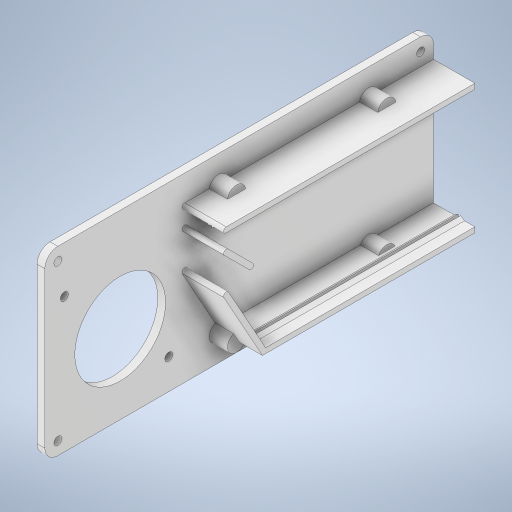
# Autodesk Inventor part: ChargingCircuit - ShroudPlate - Version2
Saved by Autodesk Inventor 2023 (Build 270158000, 158)
## iProperties
Created: 2023-01-17
Part Number: ChargingCircuit - ShroudPlate - Version2
Material: ABS Plastic
Document SubType Name: Modeling
Designer: ethan
Density: 1.06 g/cm^3
Appearance: Smooth - White
Author: ethan
Autodesk Inventor part; units mm, degrees
ref_plane "YZ Plane" through (0, 0, 0) normal (1, 0, 0) x (0, 1, 0)
ref_plane "XZ Plane" through (0, 0, 0) normal (0, 1, 0) x (-1, 0, 0)
ref_plane "XY Plane" through (0, 0, 0) normal (0, 0, 1) x (1, 0, 0)
sketch "Sketch1" plane through (0, 0, 0) normal (0, 0, 1) x (1, 0, 0)
  line L0 (0, 0) -> (150, 0)
  line L1 (150, 0) -> (150, 70)
  line L2 (150, 70) -> (0, 70)
  line L3 (0, 70) -> (0, 0)
  line L4 (5, 65) -> (145, 65) construction
  line L5 (145, 5) -> (5, 5) construction
  line L6 (5, 5) -> (5, 65) construction
  circle A0 centre (5, 65) radius 1.5
  circle A1 centre (5, 5) radius 1.5
  circle A2 centre (145, 5) radius 1.5
  circle A3 centre (145, 65) radius 1.5
  line L7 (102.1949, 52) -> (142.5, 52) construction
  line L8 (142.5, 52) -> (142.5, 11.6949) construction
  line L9 (142.5, 11.6949) -> (102.1949, 11.6949) construction
  line L10 (102.1949, 11.6949) -> (102.1949, 52) construction
  circle A4 centre (102.1949, 11.6949) radius 1.5
  circle A5 centre (142.5, 52) radius 1.5
  line L11 (102.1949, 11.6949) -> (142.5, 52) construction
  circle A6 centre (120.9332, 30.4332) radius 17.5
  line L12 (144, 53.5) -> (100.6949, 53.5) construction
  line L13 (100.6949, 53.5) -> (100.6949, 10.1949) construction
  line L14 (100.6949, 10.1949) -> (144, 10.1949) construction
  line L15 (144, 10.1949) -> (144, 53.5) construction
  line L16 (0, 56.6525) -> (0, 58.6525)
  line L17 (100.6949, 53.5) -> (100.6949, 35.6525) construction
  dimension "d0" = 150
  dimension "d1" = 70
  dimension "d2" = 5
  dimension "d3" = 5
  dimension "d4" = 60
  dimension "d5" = 140
  dimension "d6" = 3
  dimension "d7" = 3
  dimension "d8" = 3
  dimension "d9" = 3
  dimension "d13" = 40.3051
  dimension "d14" = 40.3051
  dimension "d15" = 3
  dimension "d16" = 3
  dimension "d18" = 35
  dimension "d48" = 18
  dimension "d49" = 7.5
  dimension "d50" = 18.7383
  constraints: 36 end point, 7 centre point, 7 parallel, 6 coincident, 4 horizontal, 4 tangent, 3 perpendicular, 3 point on line
  measures "d0" distance of L2.end L1.end
  measures "d1" distance of L1.end L0.end
  measures "d2" distance between parallel lines of L2 L4
  measures "d3" distance between parallel lines of L3 L6
  measures "d4" distance of L4.end L5.start
  measures "d5" distance of L4.start L4.end
  measures "d6" diameter of A0
  measures "d7" diameter of A1
  measures "d8" diameter of A2
  measures "d9" diameter of A3
  measures "d13" distance of L9.end L7.start
  measures "d14" distance of L7.start L7.end
  measures "d15" diameter of A4
  measures "d16" diameter of A5
  measures "d18" diameter of A6
  measures "d48" distance from line of L11.end L2
  measures "d49" distance from line of L1 L7.end
  measures "d50" horizontal distance of A6.centre L9.end
extrude "Extrusion1" add sketch "Sketch1" along normal blind 3
fillet "Fillet1" radius 5 4 edges at (0, 70, 1.5) (0, 0, 1.5) (150, 0, 1.5) (150, 70, 1.5)
sketch "Sketch2" plane through (0, 0, 0) normal (0, 0, -1) x (-1, 0, 0)
  line L0 (-150, 60) -> (-97, 60)
  line L1 (-150, 5) -> (-150, 65) projected
  line L2 (0, 65) -> (0, 5) projected
  line L3 (-145, 70) -> (-5, 70) projected
  line L4 (-97, 60) -> (-97, 0)
  line L5 (-5, 0) -> (-145, 0) projected
  line L6 (-97, 37) -> (-82, 10)
  line L7 (-82, 10) -> (0, 10)
  line L8 (0, 65) -> (0, 5) projected
  line L9 (-97, 41.1183) -> (-80.8232, 12)
  line L10 (-80.8232, 12) -> (0, 12)
  line L11 (-97, 60) -> (0, 60)
  line L12 (-97, 58) -> (0, 58)
  line L13 (0, 60) -> (0, 58)
  line L14 (0, 12) -> (0, 10)
  line L15 (-97, 51.1183) -> (-86.3934, 40.5117)
  line L16 (-97, 53.9467) -> (-84.9792, 41.9259)
  line L17 (-86.3934, 40.5117) -> (-84.9792, 41.9259)
  point P0 (0, 0)
  point P1 (0, 12)
  point P2 (0, 10)
  point P3 (-98, 58)
  point P4 (0, 58)
  dimension "d31" = 10
  dimension "d32" = 53
  dimension "d33" = 23
  dimension "d35" = 15
  dimension "d36" = 10
  dimension "d37" = 2
  dimension "d38" = 2
  dimension "d41" = 2
  dimension "d44" = 10
  dimension "d51" = 15
  dimension "d52" = 45
  dimension "d72" = 2
  constraints: 26 end point, 9 point on line, 3 horizontal, 3 parallel, 2 perpendicular, 2 vertical
  measures "d31" distance between parallel lines of L0 L3
  measures "d32" distance between parallel lines of L4 L1
  measures "d33" distance from line of L0 L6.start
  measures "d35" distance from line of L4 L6.end
  measures "d36" distance between parallel lines of L5 L7
  measures "d37" distance between parallel lines of L6 L9
  measures "d38" distance between parallel lines of L11 L12
  measures "d41" distance between parallel lines of L7 L10
  measures "d44" distance of L9.start L15.start
  measures "d51" distance of L15.start L15.end
  measures "d52" angle of L15 L4
  measures "d72" distance between parallel lines of L16 L15
extrude "Extrusion3" add sketch "Sketch2" along normal blind 16 contours L2 L12 L4 L11 | L2 L7 L6 L4 L9 L10 | L16 L17 L15 L4
fillet "Fillet2" radius 1 8 edges at (97, 41.1183, -8) (97, 60, -8) (97, 58, -8) (97, 37, -8) (97, 51.1183, -8) (97, 53.9467, -8) (84.9792, 41.9259, -8) (86.3934, 40.5117, -8)
sketch "Sketch3" plane through (0, 0, 3) normal (0, 0, 1) x (1, 0, 0)
  line L0 (25, 59.5) -> (83, 59.5) construction
  line L1 (83, 59.5) -> (83, 10.5) construction
  line L2 (83, 10.5) -> (25, 10.5) construction
  line L3 (25, 10.5) -> (25, 59.5) construction
  line L4 (5, 0) -> (145, 0) construction
  line L5 (145, 70) -> (5, 70) construction
  line L6 (1.5, 63) -> (86.5, 63) construction
  line L7 (86.5, 63) -> (86.5, 7) construction
  line L8 (86.5, 7) -> (1.5, 7) construction
  line L9 (1.5, 7) -> (1.5, 63) construction
  circle A0 centre (25, 10.5) radius 1.25
  circle A1 centre (25, 59.5) radius 1.25
  circle A2 centre (83, 59.5) radius 1.25
  circle A3 centre (83, 10.5) radius 1.25
  line L10 (0, 65) -> (0, 5) projected
  circle A4 centre (25, 59.5) radius 3.5
  circle A5 centre (83, 59.5) radius 3.5
  circle A6 centre (83, 10.5) radius 3.5
  circle A7 centre (25, 10.5) radius 3.5
  point P0 (0, 0)
  dimension "d53" = 58
  dimension "d54" = 49
  dimension "d55" = 70
  dimension "d56" = 10.5
  dimension "d57" = 85
  dimension "d58" = 56
  dimension "d59" = 3.5
  dimension "d61" = 2.5
  dimension "d62" = 2.5
  dimension "d63" = 2.5
  dimension "d64" = 2.5
  dimension "d70" = 1.5
  dimension "d71" = 3.5
  constraints: 16 end point, 8 centre point, 8 coincident, 4 parallel, 4 tangent, 2 horizontal, 2 perpendicular
  measures "d53" distance of L1.end L2.end
  measures "d54" distance of L0.end L1.end
  measures "d55" distance between parallel lines of L4 L5
  measures "d56" distance between parallel lines of L5 L0
  measures "d57" distance of L7.end L8.end
  measures "d58" distance of L6.end L7.end
  measures "d59" distance between parallel lines of L0 L6
  measures "d61" diameter of A0
  measures "d62" diameter of A1
  measures "d63" diameter of A2
  measures "d64" diameter of A3
  measures "d70" distance between parallel lines of L10 L9
  measures "d71" distance from line of L7 A3.centre
extrude "Extrusion5" add sketch "Sketch3" against normal blind 10 contours A0 | A1 | A2 | A3 | A4 | A5 | A6 | A7
extrude "Extrusion4" cut sketch "Sketch3" against normal blind 7 contours A0 | A1 | A2 | A3
sketch "Sketch4" plane through (0, 5, 3) normal (-1, 0, 0) x (0, 0, 1)
  line L0 (-3, 53) -> (-19, 53) projected
  line L1 (-3, 7) -> (-19, 7) projected
  line L2 (-12.5, 7) -> (-12.5, 8)
  line L3 (-12.5, 8) -> (-11, 7)
  line L4 (-13.5, 7) -> (-13.5, 8)
  line L5 (-13.5, 8) -> (-15, 7)
  line L6 (-11, 53) -> (-12.5, 53)
  line L7 (-12.5, 52) -> (-11, 53)
  line L8 (-12.5, 53) -> (-12.5, 52)
  line L9 (-13.5, 53) -> (-13.5, 52)
  line L10 (-13.5, 52) -> (-15, 53)
  line L11 (-13.5, 53) -> (-15, 53)
  line L12 (-12.5, 53) -> (-11, 53)
  line L13 (-15, 7) -> (-13.5, 7)
  line L14 (-12.5, 7) -> (-11, 7)
  point P0 (-3, -5)
  dimension "d73" = 1
  dimension "d74" = 1.5
  dimension "d75" = 1.5
  dimension "d76" = 1
  dimension "d77" = 1
  dimension "d78" = 1
  dimension "d79" = 1
  dimension "d80" = 1.5
  dimension "d81" = 1.5
  dimension "d82" = 1
  constraints: 26 end point, 4 collinear, 4 midpoint, 4 point on line, 3 vertical, 1 perpendicular
  measures "d73" distance of L2.start L2.end
  measures "d74" distance of L14.end L2.start
  measures "d75" distance of L5.end L4.start
  measures "d76" distance of L4.start L2.start
  measures "d77" distance of L6.end L8.end
  measures "d78" distance of L9.start L9.end
  measures "d79" distance of L9.start L6.end
  measures "d80" distance of point (-11, 53) L6.end
  measures "d81" distance of L10.end L9.start
  measures "d82" distance of L4.start L4.end
extrude "Extrusion6" add sketch "Sketch4" against normal up to surface contours L1 L2 L3 | L1 L5 L4 surface through (80.8232, 12, 0) normal (-0.8741573, 0.4856429, 0)
sketch "Sketch5" plane through (0, 5, 3) normal (-1, 0, 0) x (0, 0, 1)
  line L0 (-11, 7) -> (-12.5, 8) projected
  line L1 (-11, 7) -> (-11, 53)
  line L2 (-3, 53) -> (-19, 53) projected
  line L3 (-11, 53) -> (-12.5, 53)
  line L4 (-12.5, 53) -> (-12.5, 52)
  line L5 (-12.5, 52) -> (-11, 53)
  line L6 (-12.5, 53) -> (-13.5, 53)
  line L7 (-13.5, 53) -> (-13.5, 52)
  line L8 (-13.5, 52) -> (-15, 53)
  line L9 (-15, 53) -> (-13.5, 53)
  point P0 (-3, -5)
  dimension "d85" = 1.5
  dimension "d86" = 1
  dimension "d87" = 1
  dimension "d88" = 1.5
  dimension "d89" = 1
  constraints: 16 end point, 3 perpendicular, 2 point on line, 1 collinear, 1 midpoint
  measures "d85" distance of L1.end L3.end
  measures "d86" distance of L3.end L4.end
  measures "d87" distance of L3.end L6.end
  measures "d88" distance of L8.end L6.end
  measures "d89" distance of L6.end L7.end
extrude "Extrusion7" add sketch "Sketch5" against normal blind 96
equation "\"d14\" = d13"
equation "\"d41\" = d37"
equation "\"d56\" = -0.5 * d54 + 0.5 * d55"
equation "\"d59\" = -0.5 * d54 + 0.5 * d58"
body "Solid1"
